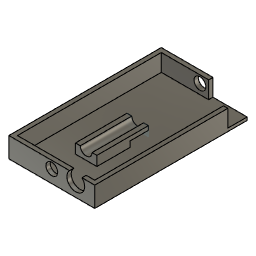
Small Magnet tray v0.3.2 (Autodesk Fusion 360 design; units mm, degrees)
Autodesk Fusion 360 part; units mm, degrees
note: some values were not read from the file. Set by a fixed rule: which sketch regions a step uses.
sketch "Sketch2" plane through (0, 0, 0) normal (0, 0, 1) x (1, 0, 0)
  line L0 (0, 0) -> (40, 0)
  line L1 (40, 0) -> (40, 71)
  line L2 (40, 71) -> (0, 71)
  line L3 (0, 71) -> (0, 0)
  line L4 (2, 2) -> (38, 2)
  line L5 (38, 2) -> (38, 69)
  line L6 (38, 69) -> (2, 69)
  line L7 (2, 69) -> (2, 2)
  dimension "d1" = 40
  dimension "d2" = 71
  dimension "d26" = 67
  constraint horizontal L0
  constraint vertical L1
  constraint horizontal L2
  constraint vertical L3
  constraint coincident L0.start L3.end
  constraint horizontal L4
  constraint vertical L5
  constraint horizontal L6
  constraint vertical L7
  measures "d1" distance of L0.start L0.end
  measures "d2" distance of L0.start L2.end
  measures "d26" distance of L4 L6
extrude "Extrude1" add sketch "Sketch2" along normal blind 9.4
sketch "Sketch3" plane through (0, 0, 0) normal (0, 0, 1) x (1, 0, 0)
  line L0 (2, 2) -> (38, 2)
  line L1 (38, 2) -> (38, 69.0002)
  line L2 (38, 69.0002) -> (2, 69.0002)
  line L3 (2, 69.0002) -> (2, 2)
  constraint horizontal L0
  constraint vertical L1
  constraint horizontal L2
  constraint vertical L3
extrude "Extrude2" add sketch "Sketch3" along normal blind 1.4
sketch "Sketch4" plane through (0, 0, 1.4) normal (0, 0, 1) x (-1, 0, 0)
  line L0 (-2, -69) -> (-2, -2)
  line L1 (-2, -2) -> (-38, -2)
  line L2 (-38, -2) -> (-38, -69)
  line L3 (-25, -30) -> (-15, -30)
  line L4 (-15, -30) -> (-15, -40)
  line L5 (-15, -40) -> (-25, -40)
  line L6 (-25, -40) -> (-25, -30)
  line L7 (-38, -69) -> (-2, -69)
  constraint horizontal L3
  constraint perpendicular L3 L4
  constraint perpendicular L4 L5
  constraint perpendicular L5 L6
extrude "Extrude3" add sketch "Sketch4" along normal blind 3 contours L3 L4 L5 L6
extrude "Extrude4" add 1 faces at (21.6667, 33.3333, 4.4) along direction (0, 0, 1) blind 1.5
hole "Hole1" at (20, 71, 5.9) direction (0, -1, 0) diameter 5.5 depth 74 tip angle 118
hole "Hole2" at (31.1767, 2, 6.3948) direction (0, -1, 0) diameter 8.3 depth 10 tip angle 118
sketch "Sketch5" plane through (0, 40, 0) normal (0, 1, 0) x (-1, 0, 0)
  arc A0 (-22.75, 5.9) -> (-17.25, 5.9) centre (-20, 5.9) ccw
  line L0 (-22.75, 5.9) -> (-25, 5.9)
  line L1 (-25, 5.9) -> (-25, 1.4)
  line L2 (-25, 1.4) -> (-15, 1.4)
  line L3 (-15, 1.4) -> (-15, 5.9)
  line L4 (-15, 5.9) -> (-17.25, 5.9)
sketch "Sketch6" plane through (0, 40, 0) normal (0, 1, 0) x (-1, 0, 0)
  line L0 (-25, 1.4) -> (-21.5733, 1.4)
  line L1 (-21.5733, 1.4) -> (-21.5733, 3.205)
  line L2 (-21.5733, 3.205) -> (-23.2867, 3.205)
  line L3 (-25, 3.205) -> (-25, 1.4)
  line L4 (-23.2867, 3.205) -> (-25, 4)
  line L5 (-25, 4) -> (-25, 3.205)
  constraint horizontal L0
  constraint vertical L1
  constraint horizontal L2
  constraint vertical L3
extrude "Extrude5" cut sketch "Sketch6" against normal blind 8.5
extrude "Extrude6" add 1 faces at (24.1592, 30, 4.0023) along direction (0, -1, 0) blind 8
sketch "Sketch7" plane through (0, 0, 9.4) normal (0, 0, 1) x (-1, 0, 0)
  line L0 (-28.3147, 0) -> (-28.3147, -2)
  line L1 (-28.3147, -2) -> (-2, -2)
  line L2 (-2, -2) -> (-2, -69)
  line L3 (-2, -69) -> (-38, -69)
  line L4 (-38, -69) -> (-38, -2)
  line L5 (-38, -2) -> (-34.0387, -2)
  line L6 (-34.0387, -2) -> (-34.0387, 0)
  line L7 (-34.0387, 0) -> (-40, 0)
  line L8 (-40, 0) -> (-40, -71)
  line L9 (-40, -71) -> (0, -71)
  line L10 (0, -71) -> (0, 0)
  line L11 (0, 0) -> (-28.3147, 0)
  line L12 (-40, -69) -> (-24.0637, -69)
  line L13 (-24.0637, -69) -> (-24.0637, -71)
  line L14 (-24.0637, -71) -> (-40, -71)
  line L15 (-40, -71) -> (-40, -69)
  constraint horizontal L12
  constraint vertical L13
  constraint horizontal L14
  constraint vertical L15
  constraint coincident L9 L13.end
  constraint coincident L8 L12.start
extrude "Extrude7" cut sketch "Sketch7" against normal blind 8 contours L3 L8 L9 L12 L13 L14 L15
sketch "Sketch8" plane through (0, 0, 9.4) normal (0, 0, 1) x (-1, 0, 0)
  line L0 (-40, -69) -> (-38, -69)
  line L1 (-38, -69) -> (-38, -2)
  line L2 (-38, -2) -> (-34.0387, -2)
  line L3 (-34.0387, -2) -> (-34.0387, 0)
  line L4 (-34.0387, 0) -> (-40, 0)
  line L5 (-40, 0) -> (-40, -69)
  line L6 (-40, -69) -> (-38, -69)
  line L7 (-38, -69) -> (-38, -62)
  line L8 (-38, -62) -> (-40, -62)
  line L9 (-40, -62) -> (-40, -69)
  constraint horizontal L6
  constraint vertical L7
  constraint horizontal L8
  constraint vertical L9
  constraint coincident L1 L7.end
  constraint coincident L0.start L5.end
extrude "Extrude8" cut sketch "Sketch8" against normal blind 8 contours L0 L1 L5 L6 L7 L8 L9
extrude "Extrude9" add 1 faces at (24.1592, 22, 4.0023) along direction (0, -1, 0) blind 6
